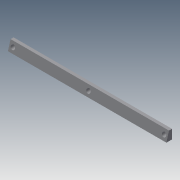
# Autodesk Inventor part: bar
Saved by Autodesk Inventor 2013 (Build 170138000, 138)
## iProperties
Created: 2013-04-24
Part Number: bar
Material: Generic
Document SubType Name: Modeling
Designer: Dave
Density: 1 g/cm^3
Author: Dave
Autodesk Inventor part; units mm, degrees
ref_plane "YZ Plane" through (0, 0, 0) normal (1, 0, 0) x (0, 1, 0)
ref_plane "XZ Plane" through (0, 0, 0) normal (0, 1, 0) x (-1, 0, 0)
ref_plane "XY Plane" through (0, 0, 0) normal (0, 0, 1) x (1, 0, 0)
sketch "Sketch1" plane through (0, 0, 0) normal (0, 0, 1) x (1, 0, 0)
  line L0 (0, 0) -> (165.1, 0)
  line L1 (165.1, 0) -> (165.1, 9.525)
  line L2 (165.1, 9.525) -> (0, 9.525)
  line L3 (0, 9.525) -> (0, 0)
  dimension "d0" = 165.1
  dimension "d1" = 9.525
  constraints: 8 end point, 2 parallel, 1 horizontal, 1 perpendicular
  measures "d0" distance of L0.start L0.end
  measures "d1" distance of L2.end L0.start
extrude "Extrusion1" add sketch "Sketch1" along normal blind 3.175
sketch "Sketch2" plane through (0, 0, 3.175) normal (0, 0, 1) x (1, 0, 0)
  line L0 (165.1, 9.525) -> (0, 9.525) projected
  line L1 (0, 9.525) -> (0, 0) projected
  circle A0 centre (3.81, 4.7625) radius 0.5592
  point P0 (82.55, 4.7625)
  point P1 (161.29, 4.7625)
  dimension "d4" = 3.81
  dimension "d5" = 4.7625
  dimension "d8" = 78.74
  constraints: 1 centre point, 1 horizontal, 2 other
  measures "d4" distance from line of L1 A0.centre
  measures "d5" distance from line of L0 A0.centre
  measures "d8" distance of A0.centre point (82.55, 4.763)
hole "Hole1" at (3.81, 4.7625, 3.175) at (82.55, 4.7625, 3.175) at (161.29, 4.7625, 3.175) direction (0, 0, -1) diameter 4.4958 end through all clearance for "Flat Head Machine Screw" size "M4" standard "Ansi Metric M Profile"
draft "FaceDraft3" angle 16 pull direction (0, 1, 0) faces at (82.55, 0.8382, 3.175) fixed edges at (82.55, 9.525, 3.175)
body "Solid1"
